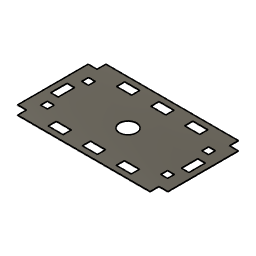
PiastraBaseScatolaGrande v6 (Autodesk Fusion 360 design; units mm, degrees)
Autodesk Fusion 360 part; units mm, degrees
note: some values were not read from the file. Chosen so that the rebuilt part matches the saved one: which face or edge a step refers to. Set by a fixed rule: which sketch regions a step uses.
sketch "Schizzo1" plane through (0, 0, 0) normal (0, 0, 1) x (1, 0, 0)
  line L0 (0, 0) -> (219.5, 0)
  line L1 (219.5, 0) -> (219.5, 129)
  line L2 (219.5, 129) -> (0, 129)
  line L3 (0, 129) -> (0, 0)
  line L4 (0, 129) -> (8.75, 129)
  line L5 (8.75, 129) -> (8.75, 0)
  line L6 (219.5, 129) -> (209.5, 129)
  line L7 (209.5, 129) -> (209.5, 0)
  line L8 (19.8077, 129) -> (19.8077, 0)
  line L9 (209.5, 64.5) -> (200, 64.5)
  line L10 (200, 129) -> (200, 0)
  line L11 (8.75, 64.5) -> (19.8077, 64.5)
  line L12 (19.8077, 64.5) -> (19.8077, 76.5)
  line L13 (19.8077, 64.5) -> (19.8077, 52.5)
  line L14 (19.8077, 76.5) -> (8.75, 76.5)
  line L15 (19.8077, 52.5) -> (8.75, 52.5)
  line L16 (0, 129) -> (17, 129)
  line L17 (17, 129) -> (17, 99.5)
  line L18 (17, 99.5) -> (27, 99.5)
  line L19 (27, 99.5) -> (27, 89.5)
  line L20 (27, 89.5) -> (17, 89.5)
  line L21 (17, 89.5) -> (17, 99.5)
  line L22 (0, 129) -> (49, 129)
  line L23 (0, 129) -> (13, 129)
  line L24 (13, 129) -> (13, 116)
  line L25 (13, 116) -> (0, 116)
  line L26 (0, 116) -> (0, 129)
  line L27 (49, 129) -> (49, 120.5)
  line L28 (49, 120.5) -> (49, 108.5)
  line L29 (49, 108.5) -> (71, 108.5)
  line L30 (71, 108.5) -> (71, 120.5)
  line L31 (71, 120.5) -> (49, 120.5)
  line L32 (0, 129) -> (98, 129)
  line L33 (98, 129) -> (98, 120.5)
  line L34 (98, 120.5) -> (98, 108.5)
  line L35 (98, 108.5) -> (120, 108.5)
  line L36 (120, 108.5) -> (120, 120.5)
  line L37 (120, 120.5) -> (98, 120.5)
  line L38 (109.75, 0) -> (109.75, 129)
  line L39 (0, 64.5) -> (219.5, 64.5)
  line L40 (8.75, 76.5) -> (8.75, 52.5)
  line L41 (199.6923, 76.5) -> (210.75, 76.5)
  line L42 (210.75, 76.5) -> (210.75, 52.5)
  line L43 (199.6923, 64.5) -> (199.6923, 76.5)
  line L44 (199.6923, 64.5) -> (199.6923, 52.5)
  line L45 (199.6923, 52.5) -> (210.75, 52.5)
  line L46 (192.5, 99.5) -> (192.5, 89.5)
  line L47 (192.5, 89.5) -> (202.5, 89.5)
  line L48 (202.5, 89.5) -> (202.5, 99.5)
  line L49 (202.5, 99.5) -> (192.5, 99.5)
  line L50 (206.5, 116) -> (219.5, 116)
  line L51 (206.5, 129) -> (206.5, 116)
  line L52 (148.5, 120.5) -> (170.5, 120.5)
  line L53 (170.5, 108.5) -> (148.5, 108.5)
  line L54 (148.5, 108.5) -> (148.5, 120.5)
  line L55 (170.5, 120.5) -> (170.5, 108.5)
  line L56 (99.5, 120.5) -> (121.5, 120.5)
  line L57 (121.5, 120.5) -> (121.5, 108.5)
  line L58 (121.5, 108.5) -> (99.5, 108.5)
  line L59 (99.5, 108.5) -> (99.5, 120.5)
  line L60 (99, 120.5) -> (99, 108.5)
  line L61 (121, 108.5) -> (121, 120.5)
  circle A0 centre (109.75, 64.5) radius 12.5
  point P0 (49, 120.5)
  point P1 (98, 120.5)
  dimension "d1" = 219.5
  dimension "d2" = 129
  dimension "d3" = 8.75
  dimension "d4" = 10
  dimension "d6" = 12
  dimension "d7" = 12
  dimension "d8" = 17
  dimension "d9" = 29.5
  dimension "d10" = 10
  dimension "d11" = 10
  dimension "d12" = 49
  dimension "d13" = 13
  dimension "d14" = 13
  dimension "d15" = 8.5
  dimension "d16" = 12
  dimension "d17" = 22
  dimension "d18" = 98
  dimension "d19" = 8.5
  dimension "d20" = 12
  dimension "d21" = 22
  dimension "d28" = 25
  constraint horizontal L0
  constraint vertical L1
  constraint horizontal L2
  constraint vertical L3
  constraint coincident L0.start L3.end
  constraint perpendicular L3 L4
  constraint coincident L0 L5.end
  constraint perpendicular L0 L5
  constraint coincident L2 L6.end
  constraint coincident L0 L7.end
  constraint perpendicular L0 L7
  constraint coincident L2 L8.start
  constraint coincident L0 L8.end
  constraint perpendicular L0 L8
  constraint midpoint L7 L9.start
  constraint perpendicular L7 L9
  constraint coincident L2 L10.start
  constraint coincident L0 L10.end
  constraint perpendicular L0 L10
  constraint midpoint L5 L11.start
  constraint midpoint L8 L11.end
  constraint coincident L8 L12.end
  constraint perpendicular L11 L12
  constraint coincident L8 L13.end
  constraint coincident L5 L14.end
  constraint perpendicular L5 L14
  constraint coincident L5 L15.end
  constraint perpendicular L5 L15
  constraint coincident L2 L16.end
  constraint perpendicular L2 L17
  constraint perpendicular L8 L18
  constraint perpendicular L18 L19
  constraint perpendicular L8 L20
  constraint perpendicular L18 L21
  constraint coincident L2 L22.end
  constraint horizontal L23
  constraint vertical L24
  constraint horizontal L25
  constraint vertical L26
  constraint perpendicular L22 L27
  constraint perpendicular L22 L28
  constraint perpendicular L28 L29
  constraint perpendicular L29 L30
  constraint perpendicular L28 L31
  constraint coincident L2 L32.end
  constraint perpendicular L32 L33
  constraint perpendicular L32 L34
  constraint perpendicular L34 L35
  constraint perpendicular L32 L36
  constraint perpendicular L33 L37
  constraint midpoint L0 L38.start
  constraint midpoint L2 L38.end
  constraint midpoint L3 L39.start
  constraint midpoint L1 L39.end
  constraint coincident P0 L27.end
  constraint coincident P1 L33.end
  constraint symmetric L11.end L38 L43.start
  constraint symmetric L12.end L38 L41.start
  constraint symmetric L13.end L38 L44.end
  constraint symmetric L14.end L38 L41.end
  constraint symmetric L15.end L38 L42.end
  constraint symmetric L17.end L38 L48.end
  constraint symmetric L18.end L38 L46.start
  constraint symmetric L19.end L38 L46.end
  constraint symmetric L20.end L38 L47.end
  constraint symmetric L23.end L38 L51.start
  constraint symmetric L24.end L38 L50.start
  constraint symmetric L25.end L38 L50.end
  constraint symmetric P0 L38 L52.end
  constraint symmetric L28.end L38 L53.start
  constraint symmetric L29.end L38 L53.end
  constraint symmetric L30.end L38 L52.start
  constraint symmetric P1 L38 L56.end
  constraint symmetric L34.end L38 L57.end
  constraint symmetric L35.end L38 L58.end
  constraint symmetric L36.end L38 L56.start
  constraint coincident L37 L60.start
  constraint coincident L35 L60.end
  constraint perpendicular L35 L60
  constraint coincident L58 L61.start
  constraint coincident L56 L61.end
  constraint perpendicular L56 L61
  constraint midpoint L38 A0.centre
  measures "d1" distance of L0.start L0.end
  measures "d2" distance of L0.start L2.end
  measures "d3" distance of L2.end L4.end
  measures "d4" distance of L1.end L6.end
  measures "d6" distance of L11.end L12.end
  measures "d7" distance of L11.end L13.end
  measures "d8" distance of L2.end L16.end
  measures "d9" distance of L16.end L17.end
  measures "d10" distance of L17.end L18.end
  measures "d11" distance of L18.end L19.end
  measures "d12" distance of L2.end L22.end
  measures "d13" distance of L2.end L23.end
  measures "d14" distance of L2.end L25.end
  measures "d15" distance of L22.end P0
  measures "d16" distance of P0 L28.end
  measures "d17" distance of L28.end L29.end
  measures "d18" distance of L2.end L32.end
  measures "d19" distance of L32.end P1
  measures "d20" distance of P1 L34.end
  measures "d21" distance of L34.end L35.end
  measures "d28" diameter of A0
extrude "Estrusione1" add sketch "Schizzo1" along normal blind 6.5 contours L3 L5 L25 L39 L40 | L2 L5 L8 L14 L16 L17 L20 L21 L22 L24 L25 L32 | L2 L8 L12 L18 L19 L20 L22 L32 L33 L34 L35 L38 L39 L58 A0 | L38 L39 A0 | L38 L39 A0 | L2 L10 L35 L37 L38 L39 L41 L43 L46 L47 L49 L56 L57 L58 A0 | L2 L8 L17 L18 L22 L32 | L1 L7 L39 L41 L42 L50 | L2 L7 L10 L41 L47 L48 L49 L50 L51 | L2 L33 L37 L38 L56 | L34 L35 L37 L60 | L56 L57 L58 L61 picked at (101.4591, 65.093) picked at (111.5169, 72.6221) makes body 1
mirror "Specchio1" about plane through (97.25, 64.5, 0) normal (0, 1, 0) of bodies 1 merged
extrude "Estrusione3" cut sketch "Schizzo1" along normal blind 2.5 contours L38 L39 A0 | L38 L39 A0 | L38 L39 A0 | L38 L39 A0 bodies 1
extrude "Estrusione4" add 1 faces at (169.0833, 64.5, 0) along direction (0, 0, -1) blind 0.5 separate body on bodies 1 makes body 2
sketch "Schizzo2" plane through (0, 0, -0.5) normal (0, 0, -1) x (1, 0, 0)
  circle A0 centre (109.75, -64.5) radius 12.5
  line L0 (19.8077, -52.5) -> (19.8077, -76.5)
  line L1 (19.8077, -76.5) -> (8.75, -76.5)
  line L2 (8.75, -76.5) -> (8.75, -52.5)
  line L3 (8.75, -52.5) -> (19.8077, -52.5)
  line L4 (0, -13) -> (0, -116)
  line L5 (0, -116) -> (13, -116)
  line L6 (13, -116) -> (13, -129)
  line L7 (13, -129) -> (206.5, -129)
  line L8 (206.5, -129) -> (206.5, -116)
  line L9 (206.5, -116) -> (219.5, -116)
  line L10 (219.5, -116) -> (219.5, -13)
  line L11 (219.5, -13) -> (206.5, -13)
  line L12 (206.5, -13) -> (206.5, 0)
  line L13 (206.5, 0) -> (13, 0)
  line L14 (13, 0) -> (13, -13)
  line L15 (13, -13) -> (0, -13)
  line L16 (27, -39.5) -> (17, -39.5)
  line L17 (17, -39.5) -> (17, -29.5)
  line L18 (17, -29.5) -> (27, -29.5)
  line L19 (27, -29.5) -> (27, -39.5)
  line L20 (121, -20.5) -> (99, -20.5)
  line L21 (99, -20.5) -> (99, -8.5)
  line L22 (99, -8.5) -> (121, -8.5)
  line L23 (121, -8.5) -> (121, -20.5)
  line L24 (192.5, -29.5) -> (202.5, -29.5)
  line L25 (202.5, -29.5) -> (202.5, -39.5)
  line L26 (202.5, -39.5) -> (192.5, -39.5)
  line L27 (192.5, -39.5) -> (192.5, -29.5)
  line L28 (49, -8.5) -> (71, -8.5)
  line L29 (71, -8.5) -> (71, -20.5)
  line L30 (71, -20.5) -> (49, -20.5)
  line L31 (49, -20.5) -> (49, -8.5)
  line L32 (148.5, -8.5) -> (170.5, -8.5)
  line L33 (170.5, -8.5) -> (170.5, -20.5)
  line L34 (170.5, -20.5) -> (148.5, -20.5)
  line L35 (148.5, -20.5) -> (148.5, -8.5)
  line L36 (170.5, -120.5) -> (148.5, -120.5)
  line L37 (148.5, -120.5) -> (148.5, -108.5)
  line L38 (148.5, -108.5) -> (170.5, -108.5)
  line L39 (170.5, -108.5) -> (170.5, -120.5)
  line L40 (71, -120.5) -> (49, -120.5)
  line L41 (49, -120.5) -> (49, -108.5)
  line L42 (49, -108.5) -> (71, -108.5)
  line L43 (71, -108.5) -> (71, -120.5)
  line L44 (202.5, -99.5) -> (192.5, -99.5)
  line L45 (192.5, -99.5) -> (192.5, -89.5)
  line L46 (192.5, -89.5) -> (202.5, -89.5)
  line L47 (202.5, -89.5) -> (202.5, -99.5)
  line L48 (99, -108.5) -> (121, -108.5)
  line L49 (121, -108.5) -> (121, -120.5)
  line L50 (121, -120.5) -> (99, -120.5)
  line L51 (99, -120.5) -> (99, -108.5)
  line L52 (17, -89.5) -> (27, -89.5)
  line L53 (27, -89.5) -> (27, -99.5)
  line L54 (27, -99.5) -> (17, -99.5)
  line L55 (17, -99.5) -> (17, -89.5)
  line L56 (199.6923, -76.5) -> (199.6923, -52.5)
  line L57 (199.6923, -52.5) -> (210.75, -52.5)
  line L58 (210.75, -52.5) -> (210.75, -76.5)
  line L59 (210.75, -76.5) -> (199.6923, -76.5)
hidden bodies 1
named bodies: "BaseScatola", "StencilDimensioni"
